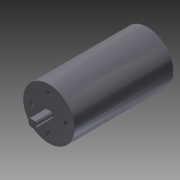
# Autodesk Inventor part: Motor
Saved by Autodesk Inventor 2014 (Build 180170000, 170)
## iProperties
Created: 2014-01-26
Part Number: Motor
Material: Aluminio-6061
Document SubType Name: Modeling
Designer: Sanjo
Density: 2.71 g/cm^3
Mass: 63.2259 g
Surface Area: 50.1281 cm^2
Volume: 23.3306 cm^3
Appearance: Acero - Pulido
Author: Sanjo
Autodesk Inventor part; units mm, degrees
ref_plane "YZ Plane" through (0, 0, 0) normal (1, 0, 0) x (0, 1, 0)
ref_plane "XZ Plane" through (0, 0, 0) normal (0, 1, 0) x (-1, 0, 0)
ref_plane "XY Plane" through (0, 0, 0) normal (0, 0, 1) x (1, 0, 0)
sketch "Boceto1" plane through (0, 0, 0) normal (0, 1, 0) x (-1, 0, 0)
  circle A0 centre (0, 0) radius 12.446
  dimension "d0" = 24.892
  constraints: 1 centre point, 1 coincident
  measures "d0" diameter of A0
extrude "Extrusión1" add sketch "Boceto1" along normal blind 48.006
sketch "Boceto2" plane through (0, 0, 0) normal (0, -1, 0) x (1, 0, 0)
  arc A0 (-1.3229, 1.5) -> (1.3229, 1.5) centre (0, 0) ccw
  line L0 (-1.3229, 1.5) -> (1.3229, 1.5)
  dimension "d3" = 4
  dimension "d4" = 1.5
  constraints: 2 end point, 2 point on circle, 1 centre point, 1 coincident, 1 horizontal
  measures "d3" diameter of A0
  measures "d4" distance from line of L0 point (0, 0)
extrude "Extrusión2" add sketch "Boceto2" along normal blind 8.001
sketch "Boceto3" plane through (0, 0, 0) normal (0, -1, 0) x (1, 0, 0)
  arc A0 (-1.3229, 1.5) -> (1.3229, 1.5) centre (0, 0) ccw projected
  point P0 (0, 8.5)
  point P1 (-8.5, 0)
  point P2 (0, -8.5)
  point P3 (8.5, 0)
  dimension "d7" = 8.5
  dimension "d10" = 360
  constraints: 5 other
  measures "d7" distance of A0.centre point (0, 8.5)
hole "Hole1" at (0, 0, 8.5) at (-8.5, 0, 0) at (0, 0, -8.5) at (8.5, 0, 0) direction (0, 1, 0) diameter 2.459 depth 6 tip angle 118 thread size "M3x0.5" class "6H" standard "ISO Metric profile"
